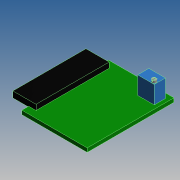
# Autodesk Inventor part: P121
Saved by Autodesk Inventor 2019 (Build 230136000, 136)
## iProperties
Created: 2017-01-25
Part Number: P121
Material: ABS Plastic
Document SubType Name: Modeling
Designer: serge.amoos
Density: 1.06 g/cm^3
Appearance: Dark Green
Description: Board laser
Author: serge.amoos
Autodesk Inventor part; units mm, degrees
ref_plane "YZ Plane" through (0, 0, 0) normal (1, 0, 0) x (0, 1, 0)
ref_plane "XZ Plane" through (0, 0, 0) normal (0, 1, 0) x (-1, 0, 0)
ref_plane "XY Plane" through (0, 0, 0) normal (0, 0, 1) x (1, 0, 0)
sketch "Sketch1" plane through (0, 0, 0) normal (0, 0, 1) x (1, 0, 0)
  line L0 (-18.76, 0) -> (18.76, 0) construction
  line L1 (0, -24.92) -> (0, 24.92) construction
  line L2 (-13.4, 17.8) -> (13.4, 17.8)
  line L3 (13.4, 17.8) -> (13.4, -17.8)
  line L4 (13.4, -17.8) -> (-13.4, -17.8)
  line L5 (-13.4, -17.8) -> (-13.4, 17.8)
  point P0 (0, 0)
  point P1 (13.4, 0)
  point P2 (0, 17.8)
  dimension "d0" = 26.8
  dimension "d1" = 35.6
  constraints: 8 end point, 2 midpoint, 2 parallel, 2 point on line, 1 horizontal, 1 perpendicular
  measures "d0" distance of L2.start L2.end
  measures "d1" distance of L2.end L3.end
extrude "Extrusion1" add sketch "Sketch1" along normal blind 1.6
sketch "Sketch3" plane through (0, 0, 1.6) normal (0, 0, 1) x (1, 0, 0)
  line L0 (5.1, 15.8) -> (11.9, 15.8)
  line L1 (11.9, 15.8) -> (11.9, 11.2)
  line L2 (11.9, 11.2) -> (5.1, 11.2)
  line L3 (5.1, 11.2) -> (5.1, 15.8)
  line L4 (13.4, 17.8) -> (-13.4, 17.8) projected
  line L5 (13.4, -17.8) -> (13.4, 17.8) projected
  point P0 (0, 0)
  dimension "d4" = 2
  dimension "d5" = 1.5
  dimension "d6" = 6.8
  dimension "d7" = 4.6
  constraints: 8 end point, 2 parallel, 1 horizontal, 1 perpendicular
  measures "d4" distance between parallel lines of L0 L4
  measures "d5" distance between parallel lines of L5 L1
  measures "d6" distance of L0.start L0.end
  measures "d7" distance of L0.end L1.end
extrude "Extrusion2" add sketch "Sketch3" along normal blind 7.3
sketch "Sketch4" plane through (0, 0, 8.9) normal (0, 0, 1) x (1, 0, 0)
  circle A0 centre (10.9, 12.2) radius 0.85
  line L0 (5.1, 11.2) -> (11.9, 11.2) projected
  line L1 (11.9, 11.2) -> (11.9, 15.8) projected
  point P0 (0, 0)
  dimension "d10" = 1.7
  dimension "d11" = 1
  dimension "d12" = 1
  constraints: 1 centre point
  measures "d10" diameter of A0
  measures "d11" distance from line of L0 A0.centre
  measures "d12" distance from line of A0.centre L1
extrude "Extrusion3" add sketch "Sketch4" along normal blind 1
sketch "Sketch5" plane through (10.9, 12.2, 9.9) normal (0, 0, 1) x (1, 0, 0)
  circle A0 centre (0, 0) radius 0.85 projected
  line L0 (-0.25, 1.1875) -> (0.25, 1.1875)
  line L1 (0.25, 1.1875) -> (0.25, -1.2526)
  line L2 (0.25, -1.2526) -> (-0.25, -1.2526)
  line L3 (-0.25, -1.2526) -> (-0.25, 1.1875)
  point P0 (-10.9, -12.2)
  point P1 (0, -1.2526)
  dimension "d15" = 0.5
  constraints: 8 end point, 2 parallel, 1 horizontal, 1 midpoint, 1 perpendicular, 1 vertical alignment
  measures "d15" distance of L0.start L0.end
extrude "Extrusion4" cut sketch "Sketch5" against normal blind 0.5 contours L1 A0 L3 | A0 L3 L0 L1 | L1 L2 L3 A0
sketch "Sketch6" plane through (0, 0, 0) normal (0, 1, 0) x (-1, 0, 0)
  line L0 (19.9, 1.3) -> (10.4, 1.3)
  line L1 (10.4, 1.3) -> (10.4, 3.8)
  line L2 (10.4, 3.8) -> (19.9, 3.8)
  line L3 (19.9, 3.8) -> (19.9, 1.3)
  line L4 (-13.4, 1.6) -> (13.4, 1.6) projected
  line L5 (13.4, 0) -> (13.4, 1.6) projected
  point P0 (0, 0)
  dimension "d18" = 0.3
  dimension "d19" = 2.5
  dimension "d20" = 6.5
  dimension "d21" = 3
  constraints: 8 end point, 2 parallel, 1 horizontal, 1 perpendicular
  measures "d18" distance between parallel lines of L4 L0
  measures "d19" distance of L0.end L1.end
  measures "d20" distance between parallel lines of L5 L3
  measures "d21" distance between parallel lines of L1 L5
extrude "Extrusion5" add sketch "Sketch6" along normal mid plane 30
equation "\"d12\" = d11"
body "Solid1"
